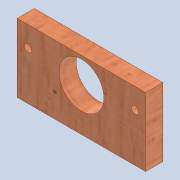
# Autodesk Inventor part: 0005-10-002 Suport1 Seringa
Saved by Autodesk Inventor 2020 (Build 240168000, 168)
## iProperties
Created: 2020-12-18
Part Number: 0005-10-002 Suport1 Seringa
Material: Generic
Document SubType Name: Modeling
Designer: Iulian Bors
Density: 1 g/cm^3
Appearance: White Oak - Natural Medium Gloss
Author: Iulian Bors
Autodesk Inventor part; units mm, degrees
ref_plane "YZ Plane" through (0, 0, 0) normal (1, 0, 0) x (0, 1, 0)
ref_plane "XZ Plane" through (0, 0, 0) normal (0, 1, 0) x (-1, 0, 0)
ref_plane "XY Plane" through (0, 0, 0) normal (0, 0, 1) x (1, 0, 0)
sketch "Sketch1" plane through (0, 0, 0) normal (0, 0, 1) x (1, 0, 0)
  line L0 (-30, 17.5) -> (30, 17.5)
  line L1 (30, 17.5) -> (30, -17.5)
  line L2 (30, -17.5) -> (-30, -17.5)
  line L3 (-30, -17.5) -> (-30, 17.5)
  point P0 (0, 0)
  point P1 (0, 17.5)
  point P2 (-30, 0)
  dimension "d0" = 60
  dimension "d1" = 35
  constraints: 8 end point, 2 midpoint, 2 parallel, 1 horizontal, 1 horizontal alignment, 1 perpendicular, 1 vertical alignment
  measures "d0" distance of L0.start L0.end
  measures "d1" distance of L2.end L0.start
extrude "Extrusion1" add sketch "Sketch1" along normal blind 8
sketch "Sketch2" plane through (0, 0, 8) normal (0, 0, 1) x (1, 0, 0)
  line L0 (0, 5) -> (0, 0) construction
  line L1 (-10.5, 5) -> (-10.5, 0)
  line L2 (10.5, 0) -> (10.5, 5)
  arc A0 (10.5, 5) -> (-10.5, 5) centre (0, 5) ccw
  arc A1 (-10.5, 0) -> (10.5, 0) centre (0, 0) ccw
  line L3 (-30, -17.5) -> (30, -17.5) projected
  line L4 (30, 17.5) -> (-30, 17.5) projected
  circle A2 centre (0, 2.5) radius 10.5
  point P0 (0, 0)
  point P1 (0, 17.5)
  dimension "d4" = 5
  dimension "d5" = 21
  dimension "d17" = 21
  dimension "d18" = 15
  constraints: 8 end point, 4 point on circle, 4 tangent, 3 centre point, 2 midpoint, 1 coincident, 1 parallel, 1 vertical, 1 vertical alignment
  measures "d4" distance of L0.start L0.end
  measures "d5" diameter of A1
  measures "d17" diameter of A2
  measures "d18" distance from line of L4 point (0, 2.5)
extrude "Extrusion2" cut sketch "Sketch2" against normal through all contours A2
sketch "Sketch3" plane through (0, 0, 8) normal (0, 0, 1) x (1, 0, 0)
  circle A0 centre (25, 5) radius 1.75
  circle A1 centre (25, 15) radius 1.75
  line L0 (30, 17.5) -> (-30, 17.5) projected
  line L1 (30, -17.5) -> (30, 17.5) projected
  circle A2 centre (-25, 5) radius 1.75
  circle A3 centre (-25, 15) radius 1.75
  line L2 (-30, 17.5) -> (-30, -17.5) projected
  point P0 (0, 0)
  dimension "d9" = 3.5
  dimension "d10" = 3.5
  dimension "d11" = 10
  dimension "d12" = 2.5
  dimension "d13" = 5
  dimension "d14" = 5
  constraints: 4 centre point, 2 equal radius, 2 horizontal alignment, 2 vertical alignment
  measures "d9" diameter of A0
  measures "d10" diameter of A1
  measures "d11" distance of A1.centre A0.centre
  measures "d12" distance from line of A1.centre L0
  measures "d13" distance from line of L1 A0.centre
  measures "d14" distance from line of A2.centre L2
extrude "Extrusion3" cut sketch "Sketch3" against normal through all contours A0 | A2
move faces "Move1" translate (0, -3, 0) faces at (10, 17.5, 2.6667)
equation "\"d14\" = d13"
body "Solid1"
